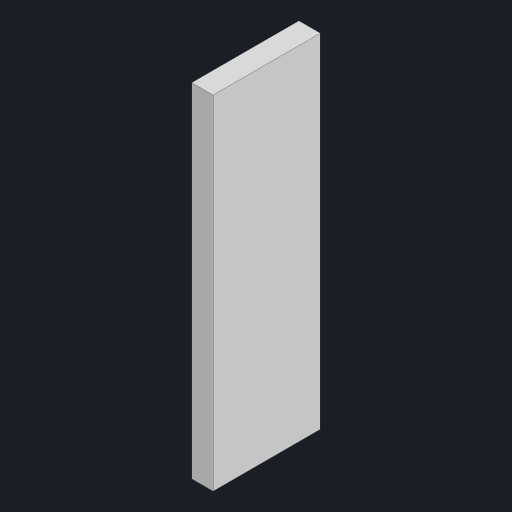
# Autodesk Inventor part: small pillar
Saved by Autodesk Inventor 2024 (Build 280153000, 153)
## iProperties
Created: 2023-11-07
Part Number: small pillar
Material: Generic
Document SubType Name: Modeling
Designer: 91840
Density: 1 g/cm^3
Appearance: Default
Author: 91840
Autodesk Inventor part; units mm, degrees
ref_plane "YZ Plane" through (0, 0, 0) normal (1, 0, 0) x (0, 1, 0)
ref_plane "XZ Plane" through (0, 0, 0) normal (0, 1, 0) x (-1, 0, 0)
ref_plane "XY Plane" through (0, 0, 0) normal (0, 0, 1) x (1, 0, 0)
sketch "Sketch1" plane through (0, 0, 0) normal (1, 0, 0) x (0, 1, 0)
  line L0 (10, 4) -> (-150, 4)
  line L1 (-150, 4) -> (-150, -46)
  line L2 (-150, -46) -> (10, -46)
  line L3 (10, -46) -> (10, 4)
  point P0 (0, 0)
  dimension "d0" = 160
  dimension "d1" = 50
  constraints: 8 end point, 2 parallel, 1 horizontal, 1 perpendicular
  measures "d0" distance of L2.end L1.end
  measures "d1" distance of L1.end L0.end
extrude "Extrusion1" add sketch "Sketch1" along normal blind 10
body "Solid1"
